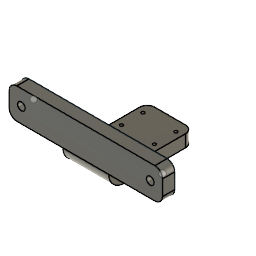
Kamera_Halterung (Autodesk Fusion 360 design; units mm, degrees)
part number: 2026-02-10-19-10-33-381
Autodesk Fusion 360 part; units mm, degrees
note: some values were not read from the file. Set by a fixed rule: which sketch regions a step uses.
sketch "Skizze1" plane through (0, 0, 0) normal (0, 0, 1) x (1, 0, 0)
  line L0 (-30, 40) -> (0, 40)
  line L1 (0, 40) -> (0, 0)
  line L2 (0, 0) -> (-30, 0)
  line L3 (-30, 0) -> (-30, 40)
  dimension "d1" = 30
  dimension "d2" = 40
  constraint horizontal L0
  constraint vertical L1
  constraint horizontal L2
  constraint vertical L3
  constraint coincident L1.end L2.start
  measures "d1" distance of L0.start L0.end
  measures "d2" distance of L0.end L1.end
extrude "Extrusion1" add sketch "Skizze1" along normal blind 8 makes body 1
sketch "Skizze2" plane through (0, 0, 8) normal (0, 0, 1) x (-1, 0, 0)
  line L0 (30, 0) -> (0, 0)
  line L1 (0, 0) -> (0, -40)
  line L2 (0, -40) -> (30, -40)
  line L3 (30, -40) -> (30, 0)
  line L4 (23, -5) -> (7, -5)
  line L5 (7, -5) -> (7, -3)
  line L6 (7, -3) -> (23, -3)
  line L7 (23, -3) -> (23, -5)
  dimension "d5" = 2
  dimension "d6" = 16
  dimension "d7" = 7
  dimension "d8" = 35
  constraint horizontal L4
  constraint vertical L5
  constraint horizontal L6
  constraint vertical L7
  measures "d5" distance of L4.start L6.end
  measures "d6" distance of L4.start L4.end
  measures "d7" distance of L3 L7
  measures "d8" distance of L2 L4
extrude "Extrusion2" cut sketch "Skizze2" against normal blind 8 contours L4 L5 L6 L7 bodies 1
sketch "Skizze3" plane through (0, 0, 0) normal (0, 0, 1) x (1, 0, 0)
ref_plane "Arbeitsebene1" through (0, 20, 4) normal (1, 0, 0) x (0, 1, 0)
sketch "Skizze4" plane through (0, 0, 0) normal (1, 0, 0) x (0, 1, 0)
  line L0 (0, 8) -> (0, 0)
  line L1 (0, 0) -> (-5, 0)
  line L2 (-15, 10) -> (-15, 30)
  arc A0 (-15, 10) -> (-5, 0) centre (-5, 10) ccw
  line L3 (-7, 10) -> (-7, 30)
  arc A1 (-7, 10) -> (-5, 8) centre (-5, 10) ccw
  line L4 (0, 8) -> (-5, 8)
  line L5 (-7, 30) -> (-15, 30)
  line L6 (0, 0) -> (-21, 0) construction
  line L7 (0, 8) -> (0, 8)
  dimension "d17" = 10
  dimension "d18" = 8
  dimension "d19" = 30
  dimension "d20" = 15
  constraint vertical L0
  constraint coincident L0.end L1.start
  constraint perpendicular L0 L1
  constraint perpendicular L1 L2
  constraint tangent L1 A0
  constraint tangent L2 A0
  constraint perpendicular L2 L5
  constraint parallel L1 L6
  measures "d17" radius of A0
  measures "d19" distance of L5 L6
  measures "d20" distance of L0 L2
extrude "Extrusion3" add sketch "Skizze4" against normal blind 30 separate body makes body 2
sketch "Skizze5" plane through (-30, 0, 0) normal (-1, 0, 0) x (0, -1, 0)
  line L0 (7, 30) -> (7, 10)
  arc A0 (5, 8) -> (7, 10) centre (5, 10) ccw
  line L1 (5, 8) -> (0, 8)
  line L2 (0, 8) -> (0, 0)
  line L3 (0, 0) -> (5, 0)
  arc A1 (5, 0) -> (15, 10) centre (5, 10) ccw
  line L4 (15, 10) -> (15, 30)
  line L5 (15, 30) -> (7, 30)
  line L6 (7, 30) -> (15, 30)
  line L7 (15, 30) -> (15, 10)
  line L8 (15, 10) -> (7, 10)
  line L9 (7, 10) -> (7, 30)
  constraint horizontal L6
  constraint vertical L7
  constraint horizontal L8
  constraint vertical L9
  constraint coincident A1.end L4.start
  constraint coincident L0.start L5.end
extrude "Extrusion4" add sketch "Skizze5" along normal blind 35 contours L0 L4 L5 L6 L7 L8 L9 bodies 2
sketch "Skizze6" plane through (0, 0, 0) normal (1, 0, 0) x (0, 1, 0)
  line L0 (-7, 10) -> (-7, 30)
  line L1 (-7, 30) -> (-15, 30)
  line L2 (-15, 30) -> (-15, 10)
  arc A0 (-15, 10) -> (-5, 0) centre (-5, 10) ccw
  line L3 (-5, 0) -> (0, 0)
  line L4 (0, 0) -> (0, 8)
  line L5 (0, 8) -> (-5, 8)
  arc A1 (-7, 10) -> (-5, 8) centre (-5, 10) ccw
  line L6 (-15, 30) -> (-7, 30)
  line L7 (-7, 30) -> (-7, 10)
  line L8 (-7, 10) -> (-15, 10)
  line L9 (-15, 10) -> (-15, 30)
  constraint horizontal L6
  constraint vertical L7
  constraint horizontal L8
  constraint vertical L9
  constraint coincident L0.start A1.start
  constraint coincident L1.end L2.start
extrude "Extrusion5" add sketch "Skizze6" along normal blind 35 contours L0 L1 L2 L6 L7 L8 L9 bodies 2
sketch "Skizze7" plane through (0, -7, 0) normal (0, 1, 0) x (-1, 0, 0)
  line L0 (0, 10) -> (30, 10)
  line L1 (30, 10) -> (65, 10)
  line L2 (65, 10) -> (65, 30)
  line L3 (65, 30) -> (-35, 30)
  line L4 (-35, 30) -> (-35, 10)
  line L5 (-35, 10) -> (0, 10)
  point P0 (-27, 20)
  point P1 (57, 20)
  dimension "d25" = 84
  dimension "d26" = 8
  measures "d25" distance of P0 P1
  measures "d26" distance of L4 P0
hole "Bohrung1" at (27, -7, 20) direction (0, -1, 0) diameter 5 depth 31 tip angle 118 bodies 2
hole "Bohrung2" at (-57, -7, 20) direction (0, -1, 0) diameter 5 depth 31 tip angle 118 bodies 2
sketch "Skizze8" plane through (0, 0, 0) normal (0, 0, -1) x (1, 0, 0)
  line L0 (-7, -3) -> (-7, -5)
  line L1 (-7, -5) -> (-23, -5)
  line L2 (-23, -5) -> (-23, -3)
  line L3 (-23, -3) -> (-7, -3)
  line L4 (0, 0) -> (-30, 0)
  line L5 (-30, 0) -> (-30, -40)
  line L6 (-30, -40) -> (0, -40)
  line L7 (0, -40) -> (0, 0)
  point P0 (-4.25, -33)
  point P1 (-25.75, -33)
  point P2 (-4.25, -19)
  point P3 (-25.75, -19)
  dimension "d33" = 21.5
  dimension "d34" = 21.5
  dimension "d35" = 14
  dimension "d36" = 4.25
  measures "d33" distance of P0 P1
  measures "d34" distance of P2 P3
  measures "d35" distance of P1 P3
  measures "d36" distance of L7 P0
hole "Bohrung3" at (-4.25, 33, 0) at (-25.75, 33, 0) at (-25.75, 19, 0) at (-4.25, 19, 0) direction (0, 0, 1) diameter 2 depth 31 tip angle 118 bodies 1
fillet "Abrundung1" radius 5 6 edges at (-30, 40, 4) (0, 40, 4) (35, -11, 10) (-65, -11, 10) (-65, -11, 30) (35, -11, 30) on bodies 1 2
